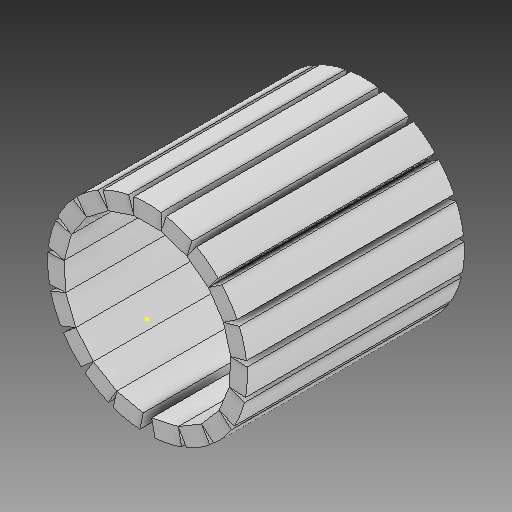
# Autodesk Inventor part: XPS
Saved by Autodesk Inventor 2021 (Build 250183000, 183)
## iProperties
Created: 2022-02-22
Part Number: XPS
Material: Generisch
Document SubType Name: Modeling
Designer: lukas
Density: 1 g/cm^3
Appearance: Vorgabe
Stock Number: XPS
Author: lukas
Autodesk Inventor part; units mm, degrees
ref_plane "YZ Plane" through (0, 0, 0) normal (1, 0, 0) x (0, 1, 0)
ref_plane "XZ Plane" through (0, 0, 0) normal (0, 1, 0) x (-1, 0, 0)
ref_plane "XY Plane" through (0, 0, 0) normal (0, 0, 1) x (1, 0, 0)
sketch "Skizze1" plane through (0, 0, 0) normal (0, 0, 1) x (1, 0, 0)
  line L0 (-257.6, 0) -> (257.6, 0) projected
  line L1 (0, -257.6) -> (0, 257.6) projected
  circle A0 centre (0, 0) radius 184
  line L2 (-25, 182.2933) -> (-25, 152.2933)
  line L3 (-25, 152.2933) -> (25, 152.2933)
  line L4 (25, 152.2933) -> (25, 182.2933)
  arc A1 (25, 182.2933) -> (-25, 182.2933) centre (0, 0.0397) ccw
  dimension "d11" = 368
  dimension "d13" = 25
  dimension "d15" = 50
  constraints: 6 end point, 2 centre point, 2 perpendicular, 2 point on circle, 1 coincident, 1 vertical
  measures "d11" diameter of A0
  measures "d13" distance from line of L1 L2.start
  measures "d15" distance between parallel lines of L4 L2
extrude "Extrusion1" add sketch "Skizze1" against normal blind 400 contours A0 L1 L3 L2 | L1 A0 L4 L3
sketch "Skizze2" plane through (0, 0, 0) normal (0, 0, 1) x (1, 0, 0)
  circle A0 centre (0, 0) radius 184
  arc A1 (25, 182.2933) -> (-25, 182.2933) centre (0, 0.0397) ccw projected
  line L0 (-25, 152.2933) -> (-25, 182.2933) projected
  arc A2 (25, 182.2933) -> (-25, 182.2933) centre (0, 0.0397) ccw
  line L1 (-25, 182.2933) -> (-25, 152.2933)
  line L2 (25, 152.2933) -> (-25, 152.2933) projected
  line L3 (25, 152.2933) -> (25, 182.2933)
  line L4 (-25, 152.2933) -> (-72.3761, 136.3088)
  line L5 (-72.3761, 136.3088) -> (-81.9668, 164.7345)
  line L6 (-25, 152.2933) -> (-34.5884, 180.7198)
  line L7 (25, 152.2933) -> (72.3761, 136.3088)
  line L8 (72.3761, 136.3088) -> (81.9668, 164.7345)
  line L9 (25, 152.2933) -> (34.5884, 180.7198)
  line L10 (72.3761, 136.3088) -> (112.1554, 106.0167)
  line L11 (112.1554, 106.0167) -> (130.3306, 129.8843)
  line L12 (72.3761, 136.3088) -> (90.5515, 160.1762)
  line L13 (-72.3761, 136.3088) -> (-112.1554, 106.0167)
  line L14 (-112.1554, 106.0167) -> (-130.3306, 129.8843)
  line L15 (-72.3761, 136.3088) -> (-90.5513, 160.1763)
  line L16 (-257.6, 0) -> (257.6, 0) projected
  line L17 (0, -257.6) -> (0, 257.6) projected
  line L18 (-112.1554, 106.0167) -> (-140.1627, 64.5971)
  line L19 (-140.1627, 64.5971) -> (-165.0145, 81.4015)
  line L20 (-112.1554, 106.0167) -> (-137.0072, 122.8212)
  line L21 (-140.1627, 64.5971) -> (-153.4585, 16.3973)
  line L22 (-153.4585, 16.3973) -> (-182.3784, 24.3747)
  line L23 (-140.1627, 64.5971) -> (-169.0826, 72.5745)
  line L24 (-153.4585, 16.3973) -> (-150.6471, -33.5236)
  line L25 (-150.6471, -33.5236) -> (-180.5996, -35.2105)
  line L26 (-153.4585, 16.3973) -> (-183.411, 14.7104)
  line L27 (-150.6471, -33.5236) -> (-132.0236, -79.9259)
  line L28 (-132.0236, -79.9259) -> (-159.8649, -91.0999)
  line L29 (-150.6471, -33.5236) -> (-178.4884, -44.6977)
  line L30 (-132.0236, -79.9259) -> (-99.5428, -117.939)
  line L31 (-99.5428, -117.939) -> (-122.3507, -137.4275)
  line L32 (-132.0236, -79.9259) -> (-154.8315, -99.4143)
  line L33 (-99.5428, -117.939) -> (-56.6139, -143.5731)
  line L34 (-56.6139, -143.5731) -> (-71.9944, -169.3305)
  line L35 (-99.5428, -117.939) -> (-114.9233, -143.6963)
  line L36 (-56.6139, -143.5731) -> (-7.7428, -154.1377)
  line L37 (-7.7428, -154.1377) -> (-14.0815, -183.4604)
  line L38 (-56.6139, -143.5731) -> (-62.9526, -172.8958)
  line L39 (112.1554, 106.0167) -> (140.1627, 64.5971)
  line L40 (140.1627, 64.5971) -> (165.0145, 81.4015)
  line L41 (112.1554, 106.0167) -> (137.0072, 122.8212)
  line L42 (140.1627, 64.5971) -> (153.4585, 16.3973)
  line L43 (153.4585, 16.3973) -> (182.3784, 24.3747)
  line L44 (140.1627, 64.5971) -> (169.0826, 72.5745)
  line L45 (153.4585, 16.3973) -> (150.6471, -33.5236)
  line L46 (150.6471, -33.5236) -> (180.5996, -35.2105)
  line L47 (153.4585, 16.3973) -> (183.411, 14.7104)
  line L48 (150.6471, -33.5236) -> (132.0236, -79.9259)
  line L49 (132.0236, -79.9259) -> (159.8649, -91.0999)
  line L50 (150.6471, -33.5236) -> (178.4884, -44.6977)
  line L51 (132.0236, -79.9259) -> (99.5428, -117.939)
  line L52 (99.5428, -117.939) -> (122.3507, -137.4275)
  line L53 (132.0236, -79.9259) -> (154.8315, -99.4143)
  line L54 (99.5428, -117.939) -> (56.6139, -143.5731)
  line L55 (56.6139, -143.5731) -> (71.9944, -169.3305)
  line L56 (99.5428, -117.939) -> (114.9233, -143.6963)
  line L57 (56.6139, -143.5731) -> (7.7428, -154.1377)
  line L58 (7.7428, -154.1377) -> (14.0815, -183.4604)
  line L59 (56.6139, -143.5731) -> (62.9526, -172.8958)
  dimension "d18" = 368
  dimension "d20" = 50
  dimension "d21" = 30
  dimension "d22" = 50
  dimension "d23" = 30
  dimension "d24" = 90
  dimension "d25" = 90.005
  dimension "d26" = 90.005
  dimension "d27" = 50
  dimension "d28" = 30
  dimension "d29" = 90
  dimension "d30" = 90
  dimension "d31" = 50
  dimension "d32" = 30
  dimension "d34" = 90
  dimension "d35" = 90
  dimension "d37" = 50
  dimension "d38" = 30
  dimension "d40" = 90
  dimension "d41" = 90
  dimension "d42" = 50
  dimension "d43" = 30
  dimension "d44" = 90
  dimension "d52" = 50
  dimension "d53" = 30
  dimension "d54" = 90
  dimension "d55" = 50
  dimension "d56" = 30
  dimension "d57" = 90
  dimension "d58" = 90
  dimension "d59" = 50
  dimension "d60" = 30
  dimension "d61" = 90
  dimension "d62" = 90
  dimension "d66" = 50
  dimension "d67" = 30
  dimension "d68" = 90
  dimension "d69" = 50
  dimension "d70" = 30
  dimension "d71" = 90
  dimension "d72" = 90
  constraints: 112 end point, 21 symmetric about line, 5 perpendicular, 2 point on circle, 1 centre point, 1 coincident, 1 collinear, 24 other
  measures "d20" distance of L0.start L4.end
  measures "d21" distance of L4.end L5.end
  measures "d22" distance of L2.start L7.end
  measures "d23" distance of L7.end L8.end
  measures "d24" angle of L7 L8
  measures "d25" angle of L7 L9
  measures "d26" angle of L4 L6
  measures "d27" distance of L7.end L10.end
  measures "d28" distance of L10.end L11.end
  measures "d29" angle of L11 L10
  measures "d30" angle of L10 L12
  measures "d31" distance of L4.end L13.end
  measures "d32" distance of L13.end L14.end
  measures "d34" angle of L13 L14
  measures "d35" angle of L13 L15
  measures "d37" distance of L13.end L18.end
  measures "d38" distance of L18.end L19.end
  measures "d40" angle of L18 L19
  measures "d41" angle of L18 L20
  measures "d42" distance of L18.end L21.end
  measures "d43" distance of L21.end L22.end
  measures "d44" angle of L21 L23
  measures "d52" distance of L21.end L24.end
  measures "d53" distance of L24.end L25.end
  measures "d54" angle of L24 L26
  measures "d55" distance of L24.end L27.end
  measures "d56" distance of L27.end L28.end
  measures "d57" angle of L28 L27
  measures "d58" angle of L27 L29
  measures "d59" distance of L27.end L30.end
  measures "d60" distance of L30.end L31.end
  measures "d61" angle of L30 L31
  measures "d62" angle of L30 L32
  measures "d66" distance of L30.end L33.end
  measures "d67" distance of L33.end L34.end
  measures "d68" angle of L33 L35
  measures "d69" distance of L33.end L36.end
  measures "d70" distance of L36.end L37.end
  measures "d71" angle of L36 L37
  measures "d72" angle of L36 L38
extrude "Extrusion2" add sketch "Skizze2" against normal blind 400 contours L16 L45 L47 A0 | A0 L46 L45 L16 | L43 L42 L44 A0 | A0 L49 L48 L50 | L39 L41 A0 L40 | L53 A0 L52 L51 | L24 L25 A0 L16 | L16 A0 L26 L24 | L10 L12 A0 L11 | L56 A0 L55 L54 | L22 A0 L23 L21 | L27 L28 A0 L29 | A0 L38 L36 L37 | L58 L57 L59 A0 | L9 A0 L8 L7 | L4 L5 A0 L6 | L19 A0 L20 L18 | L30 L31 A0 L32 | L13 L14 A0 L15 | L33 L34 A0 L35
sketch "Skizze3" plane through (0, 0, 0) normal (0, 0, 1) x (1, 0, 0)
  point P0 (0, 0)
